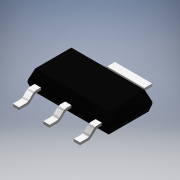
# Autodesk Inventor part: AMS1117
Saved by Autodesk Inventor 2017 SP1 (Build 210196100, 196)
## iProperties
Created: 2016-08-04
Part Number: AMS1117
Material: Generisch
Document SubType Name: Modeling
Designer: Gabriel
Density: 1 g/cm^3
Appearance: Vorgabe
Author: Gabriel
Autodesk Inventor part; units mm, degrees
ref_plane "YZ Plane" through (0, 0, 0) normal (1, 0, 0) x (0, 1, 0)
ref_plane "XZ Plane" through (0, 0, 0) normal (0, 1, 0) x (-1, 0, 0)
ref_plane "XY Plane" through (0, 0, 0) normal (0, 0, 1) x (1, 0, 0)
sketch "Skizze1" plane through (0, 0, 0) normal (0, 0, 1) x (1, 0, 0)
  line L0 (-3.25, -1.75) -> (3.25, -1.75)
  line L1 (3.25, -1.75) -> (3.25, 1.75)
  line L2 (3.25, 1.75) -> (-3.25, 1.75)
  line L3 (-3.25, 1.75) -> (-3.25, -1.75)
  line L4 (-3.25, -1.75) -> (3.25, 1.75) construction
  line L5 (3.25, -1.75) -> (-3.25, 1.75) construction
  point P0 (0, 0)
  dimension "d0" = 6.5
  dimension "d1" = 3.5
  constraints: 12 end point, 2 midpoint, 2 parallel, 1 horizontal, 1 perpendicular
  measures "d0" distance of L2.end L1.end
  measures "d1" distance of L1.end L0.end
extrude "Extrusion1" add sketch "Skizze1" along normal blind 1.5
sketch "Skizze2" plane through (3.25, -1.75, 0) normal (1, 0, 0) x (0, 0, -1)
  line L0 (0, 3.5) -> (-1.5, 3.5) projected
  line L1 (-0.7, 3.5) -> (-0.7, 4.0328)
  line L2 (-0.7, 4.0328) -> (-0.2, 4.5328)
  line L3 (-0.2, 4.5328) -> (-0.2, 5.25)
  line L4 (-0.2, 5.25) -> (0, 5.25)
  line L5 (0, 5.25) -> (0, 4.45)
  line L6 (0, 4.45) -> (-0.5, 3.95)
  line L7 (-0.5, 3.95) -> (-0.5, 3.5)
  line L8 (0, 0) -> (0, 3.5) projected
  point P0 (0, 1.75)
  dimension "d4" = 0.8
  dimension "d5" = 0.7
  dimension "d6" = 0.2
  dimension "d7" = 0.2
  dimension "d8" = 0.2
  dimension "d9" = 1.75
  dimension "d10" = 45
  constraints: 14 end point, 3 parallel, 3 perpendicular, 2 point on line, 1 collinear
  measures "d4" distance of L4.end L5.end
  measures "d5" distance between parallel lines of L8 L1
  measures "d6" distance of L3.end L4.end
  measures "d7" distance between parallel lines of L2 L6
  measures "d8" distance between parallel lines of L1 L7
  measures "d9" distance between parallel lines of L0 L4
  measures "d10" angle of L0 L6
extrude "Extrusion2" add sketch "Skizze2" against normal blind 6.5
mirror "Spiegeln1" about plane through (0, 0, 0) normal (0, 1, 0) of "Extrusion2"
sketch "Skizze3" plane through (0, 0, 1.5) normal (0, 0, 1) x (1, 0, 0)
  line L0 (-3.25, 3.5) -> (-1.5, 3.5)
  line L1 (-1.5, 3.5) -> (-1.5, 1.75)
  line L2 (-1.5, 1.75) -> (-3.25, 1.75)
  line L3 (-3.25, 1.75) -> (-3.25, 3.5)
  line L4 (1.5, 3.5) -> (3.25, 3.5)
  line L5 (3.25, 3.5) -> (3.25, 1.75)
  line L6 (3.25, 1.75) -> (1.5, 1.75)
  line L7 (1.5, 1.75) -> (1.5, 3.5)
  line L8 (-3.25, -3.5) -> (-2.7, -3.5)
  line L9 (-2.7, -3.5) -> (-2.7, -1.75)
  line L10 (-2.7, -1.75) -> (-3.25, -1.75)
  line L11 (-3.25, -1.75) -> (-3.25, -3.5)
  line L12 (-0.25, -3.5) -> (-2.2, -3.5)
  line L13 (-2.2, -3.5) -> (-2.2, -1.75)
  line L14 (-2.2, -1.75) -> (-0.25, -1.75)
  line L15 (-0.25, -1.75) -> (-0.25, -3.5)
  line L16 (0.25, -1.75) -> (2.2, -1.75)
  line L17 (2.2, -1.75) -> (2.2, -3.5)
  line L18 (2.2, -3.5) -> (0.25, -3.5)
  line L19 (0.25, -3.5) -> (0.25, -1.75)
  line L20 (2.7, -3.5) -> (3.25, -3.5)
  line L21 (3.25, -3.5) -> (3.25, -1.75)
  line L22 (3.25, -1.75) -> (2.7, -1.75)
  line L23 (2.7, -1.75) -> (2.7, -3.5)
  line L24 (-3.25, -1.75) -> (3.25, -1.75) projected
  line L25 (3.25, 3.5) -> (-3.25, 3.5) projected
  line L26 (3.25, 1.75) -> (-3.25, 1.75) projected
  line L27 (3.25, 3.5) -> (3.25, 2.7828) projected
  line L28 (-3.25, 2.7828) -> (-3.25, 3.5) projected
  line L29 (0, 5.1518) -> (0, -6.0635) construction
  line L30 (3.25, -2.2828) -> (3.25, -1.75) construction
  line L31 (3.25, -3.5) -> (-3.25, -3.5) construction
  point P0 (0, 0)
  dimension "d13" = 3
  dimension "d14" = 0.5
  dimension "d15" = 5.4
  dimension "d16" = 0.5
  constraints: 50 end point, 18 perpendicular, 15 collinear, 6 horizontal, 1 point on line, 1 vertical, 5 other
  measures "d13" distance between parallel lines of L1 L7
  measures "d14" distance between parallel lines of L15 L19
  measures "d15" distance between parallel lines of L23 L9
  measures "d16" distance between parallel lines of L9 L13
extrude "Extrusion3" cut sketch "Skizze3" against normal blind 6.5 contours L0 L1 L2 L3 | L4 L5 L6 L7 | L11 L10 L9 L8 | L22 L21 L20 L23 | L16 L17 L18 L19 | L14 L15 L12 L13
chamfer "Fase1" distance 0.3 distance2 0.8 1 edges at (0, 1.75, 1.5) measured on face at (1.0833, -0.5833, 1.5)
chamfer "Fase2" distance 0.3 distance2 0.8 1 edges at (0, -1.75, 1.5) measured on face at (-1.0833, 0.3837, 1.5)
chamfer "Fase3" distance 0.5 distance2 0.15 1 edges at (0, 1.75, 0) measured on face at (0.5, 1.75, 0.1667)
chamfer "Fase4" distance 0.5 distance2 0.15 1 edges at (0, -1.75, 0) measured on face at (-0.0833, -1.75, 0.1667)
fillet "Rundung1" radius 0.4 16 edges at (2.45, -2.2828, 0.7) (2.45, -2.2, 0.5) (2.45, -2.7, 0) (2.45, -2.7828, 0.2) (0, -2.2, 0.5) (0, -2.7, 0) (0, -2.2828, 0.7) (0, -2.7828, 0.2) (-2.45, -2.2828, 0.7) (-2.45, -2.2, 0.5) (-2.45, -2.7, 0) (-2.45, -2.7828, 0.2) (0, 2.7, 0) (0, 2.7828, 0.2) (0, 2.2, 0.5) (0, 2.2828, 0.7)
chamfer "Fase5" distance 0.5 distance2 0.15 1 edges at (-3.25, 0, 0) measured on face at (-3.25, 0.4835, 0.5)
chamfer "Fase6" distance 0.5 distance2 0.15 1 edges at (3.25, 0, 0) measured on face at (3.25, -0.4835, 0.5)
chamfer "Fase7" distance 0.3 distance2 0.8 1 edges at (3.25, 0, 1.5) measured on face at (-1.0833, 0.4835, 1.5)
chamfer "Fase8" distance 0.3 distance2 0.8 1 edges at (-3.25, 0, 1.5) measured on face at (0.8833, -0.4835, 1.5)
equation "\"d8\" = d7"
